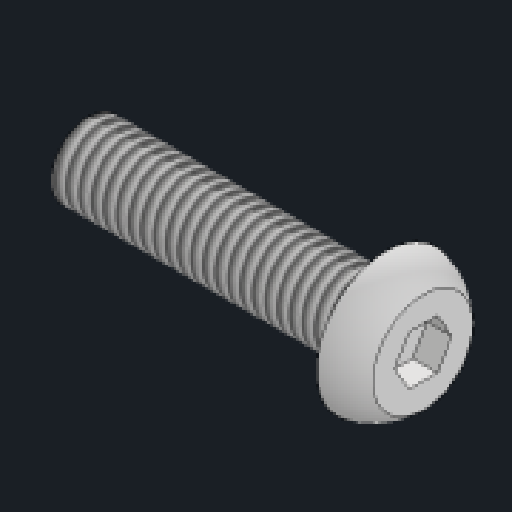
# Autodesk Inventor part: M3 x 12 Button
Saved by Autodesk Inventor 2023.2 (Build 272271030, 271C)
## iProperties
Created: 2024-02-28
Part Number: M3 x 12 Button
Material: Generic
Document SubType Name: Modeling
Designer: robpl
Density: 1 g/cm^3
Appearance: Default
Author: robpl
Autodesk Inventor part; units mm, degrees
ref_plane "YZ Plane" through (0, 0, 0) normal (1, 0, 0) x (0, 1, 0)
ref_plane "XZ Plane" through (0, 0, 0) normal (0, 1, 0) x (-1, 0, 0)
ref_plane "XY Plane" through (0, 0, 0) normal (0, 0, 1) x (1, 0, 0)
sketch "Sketch1" plane through (0, 0, 0) normal (0, 0, 1) x (1, 0, 0)
  line L0 (0, 0) -> (-12, 0)
  line L1 (-12, 0) -> (-12, 1.5)
  line L2 (-12, 1.5) -> (0, 1.5)
  line L3 (0, 1.5) -> (0, 0)
  line L4 (0, 0) -> (1.5, 0)
  line L5 (1.5, 0) -> (1.5, 2.8)
  line L6 (1.5, 2.8) -> (0, 2.8)
  line L7 (0, 2.8) -> (0, 0)
  circle A0 centre (-0.5, 0) radius 2.8443
  point P0 (1.5, 2.0224)
  dimension "d0" = 12
  dimension "d1" = 1.5
  dimension "d2" = 2.8
  dimension "d3" = 1.5
  dimension "d4" = 0.5
  constraints: 16 end point, 4 parallel, 2 horizontal, 2 perpendicular, 1 point on line, 3 other
  measures "d0" distance of L1.end L2.end
  measures "d1" distance of L0.end L1.end
  measures "d2" distance between parallel lines of L0 L6
  measures "d3" distance of L5.end L6.end
  measures "d4" distance of L0.start point (-0.5, 0)
revolve "Revolution1" add sketch "Sketch1" angle 360 about axis through (0, 0, 0) along (-1, 0, 0) contours L0 A0 L2 L3 | L3 L7 A0 L5 L4 | L0 L1 L2 A0
thread "Thread1" size "M3x0.5" class "6g" standard "ANSI Metric M Profile" full length
sketch "Sketch2" plane through (1.5, 0, 0) normal (1, 0, 0) x (0, 0, -1)
  line L0 (0.5774, 1) -> (1.1547, 0)
  line L1 (1.1547, 0) -> (0.5774, -1)
  line L2 (0.5774, -1) -> (-0.5774, -1)
  line L3 (-0.5774, -1) -> (-1.1547, 0)
  line L4 (-1.1547, 0) -> (-0.5774, 1)
  line L5 (-0.5774, 1) -> (0.5774, 1)
  point P0 (0, 0)
  point P1 (0, 0)
  point P2 (0, -1)
  dimension "d8" = 2
  constraints: 12 end point, 1 coincident, 1 horizontal, 1 midpoint, 13 other
  measures "d8" distance from line of point (0, -1) L5
extrude "Extrusion1" cut sketch "Sketch2" against normal blind 1
body "Solid1"
